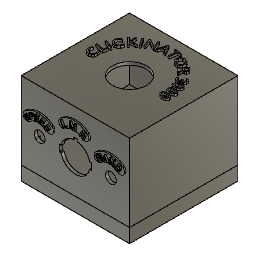
clickinator3000 v6 (Autodesk Fusion 360 design; units mm, degrees)
Autodesk Fusion 360 part; units mm, degrees
box "BoxPrimitive1" add length 70 width 70 height 50 placed x (0, 1, 0) y (-1, 0, 0) z (0, 0, 1) at (0, 0, 0) makes body 1
shell "Shell1" thickness 2 removed faces 0 bodies 1
move_body "Move1" bodies 1 to x (1, 0, 0) y (0, 1, 0) z (0, 0, 1) at (35, -35, 0)
sketch "Sketch3" plane through (0, 0, 50) normal (0, 0, 1) x (-1, 0, 0)
  line L0 (-35, -35) -> (35, -35)
  line L1 (35, -35) -> (35, 35)
  line L2 (35, 35) -> (-35, 35)
  line L3 (-35, 35) -> (-35, -35)
  circle A0 centre (0, 0) radius 11
  dimension "d7" = 22
  constraint coincident A0.centre origin
  measures "d7" diameter of A0
extrude "Extrude1" cut sketch "Sketch3" against normal up to surface (2 mm away) contours A0 bodies 1
sketch "Sketch4" plane through (0, -35, 0) normal (0, -1, 0) x (1, 0, 0)
  line L0 (-35, 50) -> (-35, 0)
  line L1 (-35, 0) -> (35, 0)
  line L2 (35, 0) -> (35, 50)
  line L3 (35, 50) -> (-35, 50)
  line L4 (0, 50) -> (0, 0) construction
  line L5 (-35, 21.8016) -> (35, 21.8016) construction
  circle A0 centre (0, 21.8016) radius 9.5
  circle A1 centre (23, 21.8016) radius 3.5
  line L6 (0, 21.8016) -> (0, 3.076) construction
  line L7 (1.1, 32.6016) -> (-1.1, 32.6016)
  line L8 (-1.1, 32.6016) -> (-1.1, 21.593)
  line L9 (-1.1, 21.593) -> (1.1, 21.593)
  line L10 (1.1, 21.593) -> (1.1, 32.6016)
  line L11 (1.1, 32.6016) -> (-1.1, 21.593) construction
  line L12 (-1.1, 32.6016) -> (1.1, 21.593) construction
  line L13 (10.4, 23.8016) -> (2.7448, 23.8016)
  line L14 (2.7448, 23.8016) -> (2.7448, 19.8016)
  line L15 (2.7448, 19.8016) -> (10.4, 19.8016)
  line L16 (10.4, 19.8016) -> (10.4, 23.8016)
  line L17 (10.4, 23.8016) -> (2.7448, 19.8016) construction
  line L18 (2.7448, 23.8016) -> (10.4, 19.8016) construction
  line L19 (0, 12.3016) -> (0, 31.3016) construction
  line L20 (-10.4, 23.8016) -> (-2.7448, 23.8016)
  line L21 (-2.7448, 19.8016) -> (-10.4, 19.8016)
  line L22 (-10.4, 19.8016) -> (-10.4, 23.8016)
  circle A2 centre (-23, 21.8016) radius 3.5
  point P0 (0, 27.0973)
  point P1 (6.5724, 21.8016)
  dimension "d10" = 19
  dimension "d12" = 7
  dimension "d14" = 2.2
  dimension "d15" = 10.8
  dimension "d16" = 4
  dimension "d17" = 10.4
  dimension "d25" = 12
  constraint midpoint L3 L4.start
  constraint coincident L4.end origin
  constraint coincident L0 L5.start
  constraint coincident L2 L5.end
  constraint perpendicular L2 L5
  constraint coincident L5 A0.centre
  constraint coincident L5 A1.centre
  constraint coincident A0.centre L6.start
  constraint perpendicular L5 L6
  constraint horizontal L7
  constraint perpendicular L7 L8
  constraint parallel L7 L9
  constraint parallel L8 L10
  constraint coincident L11 P0
  constraint coincident L12 P0
  constraint coincident L6 P0
  constraint horizontal L13
  constraint perpendicular L13 L14
  constraint parallel L13 L15
  constraint parallel L14 L16
  constraint coincident L17 P1
  constraint coincident L18 P1
  constraint coincident L5 P1
  constraint coincident L6 L19.start
  constraint coincident A0 L19.start
  constraint coincident A0 L19.end
  constraint vertical L19
  constraint symmetric L13.start L19 L20.start
  constraint symmetric L13.end L19 L20.end
  constraint symmetric L14.end L19 L21.start
  constraint symmetric L15.end L19 L21.end
  constraint coincident L4 A0.centre
  constraint symmetric L4 A1 A2
  measures "d10" diameter of A0
  measures "d12" diameter of A1
  measures "d14" distance of L8 L10
  measures "d15" distance of A0.centre L7
  measures "d16" distance of L13.end L14.end
  measures "d17" distance of A0.centre L16
  measures "d25" distance of L2 A1.centre
extrude "Extrude2" cut sketch "Sketch4" against normal up to surface (2 mm away) contours A0 L13 L14 L15 | A0 L13 L15 L16 | A0 L8 L9 L10 L13 L14 L15 | A0 L8 L9 L10 | A0 L7 L8 L10 | A0 L20 L21 L22 | A1 | A2 bodies 1
sketch "Sketch5" plane through (0, 0, 0) normal (0, 0, 1) x (1, 0, 0)
sketch "Sketch7" plane through (0, 0, 0) normal (1, 0, 0) x (0, 1, 0)
sketch "Sketch8" plane through (0, 0, 0) normal (0, 0, 1) x (1, 0, 0)
  line L0 (-22.8999, 2.8965) -> (-21.9973, 2.9285)
  spline S0 degree 2 poles (-21.9973, 2.9285) (-21.473, 2.0435) (-21.431, 0.862) knots 0 0 0 1 1 1
  spline S1 degree 2 poles (-21.431, 0.862) (-21.3969, -0.098) (-21.7588, -0.7804) knots 0 0 0 1 1 1
  spline S2 degree 2 poles (-21.7588, -0.7804) (-22.1207, -1.4628) (-22.7837, -1.8766) knots 0 0 0 1 1 1
  spline S3 degree 2 poles (-22.7837, -1.8766) (-23.4468, -2.2903) (-24.2345, -2.3183) knots 0 0 0 1 1 1
  spline S4 degree 2 poles (-24.2345, -2.3183) (-25.4857, -2.3628) (-26.3706, -1.5029) knots 0 0 0 1 1 1
  spline S5 degree 2 poles (-26.3706, -1.5029) (-27.2557, -0.6388) (-27.3022, 0.6698) knots 0 0 0 1 1 1
  spline S6 degree 2 poles (-27.3022, 0.6698) (-27.3343, 1.5724) (-26.9017, 2.6927) knots 0 0 0 1 1 1
  line L1 (-26.9017, 2.6927) -> (-26.0197, 2.724)
  spline S7 degree 2 poles (-26.0197, 2.724) (-26.5583, 1.6985) (-26.5242, 0.7386) knots 0 0 0 1 1 1
  spline S8 degree 2 poles (-26.5242, 0.7386) (-26.4892, -0.246) (-25.8425, -0.8762) knots 0 0 0 1 1 1
  spline S9 degree 2 poles (-25.8425, -0.8762) (-25.2, -1.5023) (-24.2646, -1.4691) knots 0 0 0 1 1 1
  spline S10 degree 2 poles (-24.2646, -1.4691) (-23.3211, -1.4356) (-22.7366, -0.774) knots 0 0 0 1 1 1
  spline S11 degree 2 poles (-22.7366, -0.774) (-22.1522, -0.1125) (-22.1876, 0.8844) knots 0 0 0 1 1 1
  spline S12 degree 2 poles (-22.1876, 0.8844) (-22.2246, 1.9264) (-22.8999, 2.8965) knots 0 0 0 1 1 1
  line L2 (-26.9677, 5.1045) -> (-26.8044, 5.9091)
  line L3 (-26.8044, 5.9091) -> (-21.9164, 4.9171)
  line L4 (-21.9164, 4.9171) -> (-21.4029, 7.4475)
  line L5 (-21.4029, 7.4475) -> (-20.6707, 7.2989)
  line L6 (-20.6707, 7.2989) -> (-21.3475, 3.9638)
  line L7 (-21.3475, 3.9638) -> (-26.9677, 5.1045)
  line L8 (-25.7564, 9.9218) -> (-25.4772, 10.6938)
  line L9 (-25.4772, 10.6938) -> (-20.0844, 8.7432)
  line L10 (-20.0844, 8.7432) -> (-20.3636, 7.9712)
  line L11 (-20.3636, 7.9712) -> (-25.7564, 9.9218)
  line L12 (-18.3113, 14.9034) -> (-17.536, 14.4404)
  spline S13 degree 2 poles (-17.536, 14.4404) (-17.576, 13.4124) (-18.1822, 12.3974) knots 0 0 0 1 1 1
  spline S14 degree 2 poles (-18.1822, 12.3974) (-18.6746, 11.5727) (-19.349, 11.196) knots 0 0 0 1 1 1
  spline S15 degree 2 poles (-19.349, 11.196) (-20.0233, 10.8194) (-20.8048, 10.8318) knots 0 0 0 1 1 1
  spline S16 degree 2 poles (-20.8048, 10.8318) (-21.5863, 10.8442) (-22.263, 11.2483) knots 0 0 0 1 1 1
  spline S17 degree 2 poles (-22.263, 11.2483) (-23.3379, 11.8902) (-23.6143, 13.0928) knots 0 0 0 1 1 1
  spline S18 degree 2 poles (-23.6143, 13.0928) (-23.8886, 14.2989) (-23.2173, 15.4232) knots 0 0 0 1 1 1
  spline S19 degree 2 poles (-23.2173, 15.4232) (-22.7542, 16.1986) (-21.7828, 16.9046) knots 0 0 0 1 1 1
  line L13 (-21.7828, 16.9046) -> (-21.025, 16.4521)
  spline S20 degree 2 poles (-21.025, 16.4521) (-22.0341, 15.8833) (-22.5266, 15.0586) knots 0 0 0 1 1 1
  spline S21 degree 2 poles (-22.5266, 15.0586) (-23.0317, 14.2127) (-22.8306, 13.3324) knots 0 0 0 1 1 1
  spline S22 degree 2 poles (-22.8306, 13.3324) (-22.6309, 12.4577) (-21.8273, 11.9779) knots 0 0 0 1 1 1
  spline S23 degree 2 poles (-21.8273, 11.9779) (-21.0167, 11.4938) (-20.1668, 11.7322) knots 0 0 0 1 1 1
  spline S24 degree 2 poles (-20.1668, 11.7322) (-19.3168, 11.9705) (-18.8054, 12.8269) knots 0 0 0 1 1 1
  spline S25 degree 2 poles (-18.8054, 12.8269) (-18.2708, 13.7222) (-18.3113, 14.9034) knots 0 0 0 1 1 1
  line L14 (-18.0809, 21.3843) -> (-17.3385, 22.0929)
  line L15 (-17.3385, 22.0929) -> (-17.2619, 18.4095)
  line L16 (-17.2619, 18.4095) -> (-12.9367, 18.3666)
  line L17 (-12.9367, 18.3666) -> (-13.7504, 17.59)
  line L18 (-13.7504, 17.59) -> (-17.8233, 17.6183)
  line L19 (-17.8233, 17.6183) -> (-15.8677, 15.5693)
  line L20 (-15.8677, 15.5693) -> (-16.4616, 15.0024)
  line L21 (-16.4616, 15.0024) -> (-20.421, 19.151)
  line L22 (-20.421, 19.151) -> (-19.827, 19.7178)
  line L23 (-19.827, 19.7178) -> (-18.016, 17.8202)
  line L24 (-18.016, 17.8202) -> (-18.0809, 21.3843)
  line L25 (-15.4558, 23.3953) -> (-14.7707, 23.8477)
  line L26 (-14.7707, 23.8477) -> (-11.6112, 19.0618)
  line L27 (-11.6112, 19.0618) -> (-12.2964, 18.6094)
  line L28 (-12.2964, 18.6094) -> (-15.4558, 23.3953)
  line L29 (-8.4728, 26.8725) -> (-7.7482, 27.1613)
  line L30 (-7.7482, 27.1613) -> (-5.6248, 21.8342)
  line L31 (-5.6248, 21.8342) -> (-6.2807, 21.5728)
  line L32 (-6.2807, 21.5728) -> (-11.4762, 24.2523)
  line L33 (-11.4762, 24.2523) -> (-9.8422, 20.1531)
  line L34 (-9.8422, 20.1531) -> (-10.5591, 19.8673)
  line L35 (-10.5591, 19.8673) -> (-12.6826, 25.1944)
  line L36 (-12.6826, 25.1944) -> (-12.0648, 25.4407)
  line L37 (-12.0648, 25.4407) -> (-6.8251, 22.739)
  line L38 (-6.8251, 22.739) -> (-8.4728, 26.8725)
  line L39 (-3.0804, 27.9667) -> (-2.5039, 28.0191)
  line L40 (-2.5039, 28.0191) -> (0.5733, 22.5075)
  line L41 (0.5733, 22.5075) -> (-0.2648, 22.4313)
  line L42 (-0.2648, 22.4313) -> (-1.179, 24.0547)
  line L43 (-1.179, 24.0547) -> (-3.6074, 23.8339)
  line L44 (-3.6074, 23.8339) -> (-4.1731, 22.076)
  line L45 (-4.1731, 22.076) -> (-5.0111, 21.9998)
  line L46 (-5.0111, 21.9998) -> (-3.0804, 27.9667)
  line L47 (-1.5804, 24.7519) -> (-2.6883, 26.7369)
  line L48 (-2.6883, 26.7369) -> (-3.3547, 24.5906)
  line L49 (-3.3547, 24.5906) -> (-1.5804, 24.7519)
  line L50 (1.6645, 28.1176) -> (6.394, 27.3551)
  line L51 (6.394, 27.3551) -> (6.2777, 26.6337)
  line L52 (6.2777, 26.6337) -> (4.304, 26.9519)
  line L53 (4.304, 26.9519) -> (3.5062, 22.0035)
  line L54 (3.5062, 22.0035) -> (2.6916, 22.1348)
  line L55 (2.6916, 22.1348) -> (3.4894, 27.0832)
  line L56 (3.4894, 27.0832) -> (1.5482, 27.3961)
  line L57 (1.5482, 27.3961) -> (1.6645, 28.1176)
  spline S26 degree 2 poles (11.3054, 25.5557) (12.5069, 24.9854) (12.9434, 23.8467) knots 0 0 0 1 1 1
  spline S27 degree 2 poles (12.9434, 23.8467) (13.3835, 22.7062) (12.8396, 21.5603) knots 0 0 0 1 1 1
  spline S28 degree 2 poles (12.8396, 21.5603) (12.2957, 20.4144) (11.1299, 20.0453) knots 0 0 0 1 1 1
  spline S29 degree 2 poles (11.1299, 20.0453) (9.9696, 19.6782) (8.7421, 20.2608) knots 0 0 0 1 1 1
  spline S30 degree 2 poles (8.7421, 20.2608) (7.5702, 20.8171) (7.1433, 21.9376) knots 0 0 0 1 1 1
  spline S31 degree 2 poles (7.1433, 21.9376) (6.7219, 23.0601) (7.2588, 24.1912) knots 0 0 0 1 1 1
  spline S32 degree 2 poles (7.2588, 24.1912) (7.8097, 25.3519) (8.9568, 25.739) knots 0 0 0 1 1 1
  spline S33 degree 2 poles (8.9568, 25.739) (10.1038, 26.126) (11.3054, 25.5557) knots 0 0 0 1 1 1
  spline S34 degree 2 poles (11.0006, 24.837) (10.1105, 25.2595) (9.2717, 24.9761) knots 0 0 0 1 1 1
  spline S35 degree 2 poles (9.2717, 24.9761) (8.4366, 24.6909) (8.0264, 23.8268) knots 0 0 0 1 1 1
  spline S36 degree 2 poles (8.0264, 23.8268) (7.6286, 22.9887) (7.9394, 22.1596) knots 0 0 0 1 1 1
  spline S37 degree 2 poles (7.9394, 22.1596) (8.2501, 21.3305) (9.1142, 20.9203) knots 0 0 0 1 1 1
  spline S38 degree 2 poles (9.1142, 20.9203) (9.982, 20.5084) (10.8298, 20.8012) knots 0 0 0 1 1 1
  spline S39 degree 2 poles (10.8298, 20.8012) (11.6814, 21.0923) (12.0827, 21.9378) knots 0 0 0 1 1 1
  spline S40 degree 2 poles (12.0827, 21.9378) (12.4735, 22.7611) (12.1571, 23.5974) knots 0 0 0 1 1 1
  spline S41 degree 2 poles (12.1571, 23.5974) (11.8461, 24.4357) (11.0006, 24.837) knots 0 0 0 1 1 1
  line L58 (12.4066, 18.2385) -> (16.2174, 22.5238)
  line L59 (16.2174, 22.5238) -> (17.2911, 21.5691)
  spline S42 degree 2 poles (17.2911, 21.5691) (17.9414, 20.9908) (18.0353, 20.3304) knots 0 0 0 1 1 1
  spline S43 degree 2 poles (18.0353, 20.3304) (18.1324, 19.6673) (17.6441, 19.1182) knots 0 0 0 1 1 1
  spline S44 degree 2 poles (17.6441, 19.1182) (17.3113, 18.744) (16.8814, 18.6374) knots 0 0 0 1 1 1
  spline S45 degree 2 poles (16.8814, 18.6374) (16.4515, 18.5308) (15.9817, 18.7067) knots 0 0 0 1 1 1
  spline S46 degree 2 poles (15.9817, 18.7067) (16.0672, 18.389) (16.0562, 17.9813) knots 0 0 0 1 1 1
  spline S47 degree 2 poles (16.0562, 17.9813) (16.0452, 17.5735) (15.8855, 16.6773) knots 0 0 0 1 1 1
  spline S48 degree 2 poles (15.8855, 16.6773) (15.7848, 16.1132) (15.7561, 15.8091) knots 0 0 0 1 1 1
  line L60 (15.7561, 15.8091) -> (15.7103, 15.3005)
  line L61 (15.7103, 15.3005) -> (14.9802, 15.9497)
  line L62 (14.9802, 15.9497) -> (15.0441, 16.3983)
  spline S49 degree 2 poles (15.0441, 16.3983) (15.0485, 16.4218) (15.0537, 16.4832) knots 0 0 0 1 1 1
  line L63 (15.0537, 16.4832) -> (15.0841, 16.7583)
  line L64 (15.0841, 16.7583) -> (15.1721, 17.2403)
  line L65 (15.1721, 17.2403) -> (15.2639, 17.7575)
  spline S50 degree 2 poles (15.2639, 17.7575) (15.3083, 18.1904) (15.2879, 18.4887) knots 0 0 0 1 1 1
  spline S51 degree 2 poles (15.2879, 18.4887) (15.2706, 18.7843) (15.2018, 18.9663) knots 0 0 0 1 1 1
  spline S52 degree 2 poles (15.2018, 18.9663) (15.1388, 19.1487) (14.8382, 19.4161) knots 0 0 0 1 1 1
  line L66 (14.8382, 19.4161) -> (14.6786, 19.5579)
  line L67 (14.6786, 19.5579) -> (13.0201, 17.6928)
  line L68 (13.0201, 17.6928) -> (12.4066, 18.2385)
  line L69 (16.5513, 21.2931) -> (16.3672, 21.4568)
  line L70 (16.3672, 21.4568) -> (15.1642, 20.104)
  line L71 (15.1642, 20.104) -> (15.3973, 19.8967)
  spline S53 degree 2 poles (15.3973, 19.8967) (15.8636, 19.482) (16.1063, 19.409) knots 0 0 0 1 1 1
  spline S54 degree 2 poles (16.1063, 19.409) (16.3521, 19.3332) (16.589, 19.4082) knots 0 0 0 1 1 1
  spline S55 degree 2 poles (16.589, 19.4082) (16.8318, 19.4835) (17.0145, 19.689) knots 0 0 0 1 1 1
  spline S56 degree 2 poles (17.0145, 19.689) (17.1946, 19.8915) (17.2318, 20.1495) knots 0 0 0 1 1 1
  spline S57 degree 2 poles (17.2318, 20.1495) (17.2717, 20.4107) (17.1354, 20.6527) knots 0 0 0 1 1 1
  spline S58 degree 2 poles (17.1354, 20.6527) (17.0022, 20.8921) (16.5513, 21.2931) knots 0 0 0 1 1 1
  line L72 (20.7885, 13.7546) -> (20.8128, 13.7118)
  spline S59 degree 2 poles (20.8128, 13.7118) (21.0786, 13.2443) (21.4092, 13.1112) knots 0 0 0 1 1 1
  spline S60 degree 2 poles (21.4092, 13.1112) (21.7419, 12.9745) (22.1095, 13.1835) knots 0 0 0 1 1 1
  spline S61 degree 2 poles (22.1095, 13.1835) (22.4414, 13.3721) (22.5124, 13.7289) knots 0 0 0 1 1 1
  spline S62 degree 2 poles (22.5124, 13.7289) (22.5855, 14.0821) (22.3664, 14.4675) knots 0 0 0 1 1 1
  spline S63 degree 2 poles (22.3664, 14.4675) (22.1453, 14.8565) (21.6328, 15.1932) knots 0 0 0 1 1 1
  line L73 (21.6328, 15.1932) -> (22.3144, 15.5807)
  spline S64 degree 2 poles (22.3144, 15.5807) (22.7796, 15.269) (23.0718, 14.7552) knots 0 0 0 1 1 1
  spline S65 degree 2 poles (23.0718, 14.7552) (23.4633, 14.0664) (23.3281, 13.4654) knots 0 0 0 1 1 1
  spline S66 degree 2 poles (23.3281, 13.4654) (23.1948, 12.8608) (22.5703, 12.5058) knots 0 0 0 1 1 1
  spline S67 degree 2 poles (22.5703, 12.5058) (22.192, 12.2907) (21.8443, 12.2961) knots 0 0 0 1 1 1
  spline S68 degree 2 poles (21.8443, 12.2961) (21.5001, 12.3035) (21.1238, 12.5334) knots 0 0 0 1 1 1
  spline S69 degree 2 poles (21.1238, 12.5334) (21.176, 12.1759) (21.0853, 11.9449) knots 0 0 0 1 1 1
  spline S70 degree 2 poles (21.0853, 11.9449) (20.9983, 11.716) (20.8053, 11.5071) knots 0 0 0 1 1 1
  spline S71 degree 2 poles (20.8053, 11.5071) (20.6124, 11.2983) (20.3483, 11.1482) knots 0 0 0 1 1 1
  spline S72 degree 2 poles (20.3483, 11.1482) (19.6953, 10.7769) (19.0195, 10.9688) knots 0 0 0 1 1 1
  spline S73 degree 2 poles (19.0195, 10.9688) (18.3473, 11.1628) (17.97, 11.8266) knots 0 0 0 1 1 1
  spline S74 degree 2 poles (17.97, 11.8266) (17.6474, 12.394) (17.622, 13.0784) knots 0 0 0 1 1 1
  line L74 (17.622, 13.0784) -> (18.3999, 13.5206)
  spline S75 degree 2 poles (18.3999, 13.5206) (18.3672, 12.7559) (18.6695, 12.2242) knots 0 0 0 1 1 1
  spline S76 degree 2 poles (18.6695, 12.2242) (18.8744, 11.8638) (19.2122, 11.7678) knots 0 0 0 1 1 1
  spline S77 degree 2 poles (19.2122, 11.7678) (19.5521, 11.6682) (19.9054, 11.8691) knots 0 0 0 1 1 1
  spline S78 degree 2 poles (19.9054, 11.8691) (20.2016, 12.0375) (20.3194, 12.3453) knots 0 0 0 1 1 1
  spline S79 degree 2 poles (20.3194, 12.3453) (20.3835, 12.5233) (20.3655, 12.6878) knots 0 0 0 1 1 1
  spline S80 degree 2 poles (20.3655, 12.6878) (20.3531, 12.8508) (20.1611, 13.313) knots 0 0 0 1 1 1
  line L75 (20.1611, 13.313) -> (20.1318, 13.3813)
  line L76 (20.1318, 13.3813) -> (20.7885, 13.7546)
  spline S81 degree 2 poles (25.4073, 9.5475) (25.6541, 8.799) (25.0274, 8.052) knots 0 0 0 1 1 1
  spline S82 degree 2 poles (25.0274, 8.052) (24.4058, 7.3023) (23.1972, 6.9038) knots 0 0 0 1 1 1
  spline S83 degree 2 poles (23.1972, 6.9038) (21.9575, 6.4949) (21.0197, 6.7303) knots 0 0 0 1 1 1
  spline S84 degree 2 poles (21.0197, 6.7303) (20.0832, 6.9617) (19.8261, 7.7414) knots 0 0 0 1 1 1
  spline S85 degree 2 poles (19.8261, 7.7414) (19.5651, 8.5328) (20.1671, 9.263) knots 0 0 0 1 1 1
  spline S86 degree 2 poles (20.1671, 9.263) (20.7692, 9.9933) (22.0245, 10.4073) knots 0 0 0 1 1 1
  spline S87 degree 2 poles (22.0245, 10.4073) (23.2642, 10.8161) (24.2033, 10.5769) knots 0 0 0 1 1 1
  spline S88 degree 2 poles (24.2033, 10.5769) (25.1463, 10.3389) (25.4073, 9.5475) knots 0 0 0 1 1 1
  line L77 (24.6691, 9.2954) -> (24.6563, 9.3344)
  spline S89 degree 2 poles (24.6563, 9.3344) (24.5084, 9.7828) (23.8674, 9.8653) knots 0 0 0 1 1 1
  spline S90 degree 2 poles (23.8674, 9.8653) (23.2316, 9.9452) (22.2881, 9.6341) knots 0 0 0 1 1 1
  spline S91 degree 2 poles (22.2881, 9.6341) (21.3213, 9.3152) (20.8565, 8.8766) knots 0 0 0 1 1 1
  spline S92 degree 2 poles (20.8565, 8.8766) (20.3917, 8.438) (20.5408, 7.9858) knots 0 0 0 1 1 1
  spline S93 degree 2 poles (20.5408, 7.9858) (20.69, 7.5336) (21.3258, 7.4537) knots 0 0 0 1 1 1
  spline S94 degree 2 poles (21.3258, 7.4537) (21.9616, 7.3738) (22.905, 7.6849) knots 0 0 0 1 1 1
  spline S95 degree 2 poles (22.905, 7.6849) (23.8524, 7.9973) (24.3302, 8.4359) knots 0 0 0 1 1 1
  spline S96 degree 2 poles (24.3302, 8.4359) (24.8093, 8.8705) (24.6691, 9.2954) knots 0 0 0 1 1 1
  spline S97 degree 2 poles (26.5632, 4.3205) (26.6568, 3.5379) (25.8945, 2.9298) knots 0 0 0 1 1 1
  spline S98 degree 2 poles (25.8945, 2.9298) (25.1367, 2.3182) (23.8731, 2.167) knots 0 0 0 1 1 1
  spline S99 degree 2 poles (23.8731, 2.167) (22.577, 2.0119) (21.7044, 2.4284) knots 0 0 0 1 1 1
  spline S100 degree 2 poles (21.7044, 2.4284) (20.8323, 2.8408) (20.7348, 3.656) knots 0 0 0 1 1 1
  spline S101 degree 2 poles (20.7348, 3.656) (20.6357, 4.4834) (21.3706, 5.0799) knots 0 0 0 1 1 1
  spline S102 degree 2 poles (21.3706, 5.0799) (22.1054, 5.6764) (23.4178, 5.8334) knots 0 0 0 1 1 1
  spline S103 degree 2 poles (23.4178, 5.8334) (24.714, 5.9886) (25.587, 5.568) knots 0 0 0 1 1 1
  spline S104 degree 2 poles (25.587, 5.568) (26.4642, 5.1479) (26.5632, 4.3205) knots 0 0 0 1 1 1
  line L78 (25.7897, 4.2196) -> (25.7848, 4.2604)
  spline S105 degree 2 poles (25.7848, 4.2604) (25.7287, 4.7291) (25.1168, 4.9371) knots 0 0 0 1 1 1
  spline S106 degree 2 poles (25.1168, 4.9371) (24.5094, 5.1414) (23.523, 5.0234) knots 0 0 0 1 1 1
  spline S107 degree 2 poles (23.523, 5.0234) (22.5122, 4.9024) (21.9697, 4.5646) knots 0 0 0 1 1 1
  spline S108 degree 2 poles (21.9697, 4.5646) (21.4272, 4.2268) (21.4837, 3.754) knots 0 0 0 1 1 1
  spline S109 degree 2 poles (21.4837, 3.754) (21.5403, 3.2812) (22.1477, 3.0769) knots 0 0 0 1 1 1
  spline S110 degree 2 poles (22.1477, 3.0769) (22.7551, 2.8726) (23.7415, 2.9906) knots 0 0 0 1 1 1
  spline S111 degree 2 poles (23.7415, 2.9906) (24.7319, 3.1091) (25.2872, 3.4443) knots 0 0 0 1 1 1
  spline S112 degree 2 poles (25.2872, 3.4443) (25.8429, 3.7754) (25.7897, 4.2196) knots 0 0 0 1 1 1
  spline S113 degree 2 poles (26.663, -1.0225) (26.601, -1.8083) (25.734, -2.2546) knots 0 0 0 1 1 1
  spline S114 degree 2 poles (25.734, -2.2546) (24.8707, -2.7053) (23.6021, -2.6052) knots 0 0 0 1 1 1
  spline S115 degree 2 poles (23.6021, -2.6052) (22.3008, -2.5026) (21.5271, -1.9227) knots 0 0 0 1 1 1
  spline S116 degree 2 poles (21.5271, -1.9227) (20.7531, -1.3469) (20.8176, -0.5285) knots 0 0 0 1 1 1
  spline S117 degree 2 poles (20.8176, -0.5285) (20.8832, 0.3023) (21.7209, 0.7427) knots 0 0 0 1 1 1
  spline S118 degree 2 poles (21.7209, 0.7427) (22.5586, 1.1831) (23.8763, 1.0791) knots 0 0 0 1 1 1
  spline S119 degree 2 poles (23.8763, 1.0791) (25.1777, 0.9765) (25.951, 0.3925) knots 0 0 0 1 1 1
  spline S120 degree 2 poles (25.951, 0.3925) (26.7285, -0.1918) (26.663, -1.0225) knots 0 0 0 1 1 1
  line L79 (25.8848, -0.9694) -> (25.888, -0.9284)
  spline S121 degree 2 poles (25.888, -0.9284) (25.9252, -0.4578) (25.366, -0.1337) knots 0 0 0 1 1 1
  spline S122 degree 2 poles (25.366, -0.1337) (24.8106, 0.186) (23.8203, 0.2642) knots 0 0 0 1 1 1
  spline S123 degree 2 poles (23.8203, 0.2642) (22.8054, 0.3443) (22.2071, 0.1197) knots 0 0 0 1 1 1
  spline S124 degree 2 poles (22.2071, 0.1197) (21.6087, -0.1049) (21.5713, -0.5796) knots 0 0 0 1 1 1
  spline S125 degree 2 poles (21.5713, -0.5796) (21.5338, -1.0543) (22.0892, -1.374) knots 0 0 0 1 1 1
  spline S126 degree 2 poles (22.0892, -1.374) (22.6446, -1.6937) (23.635, -1.7718) knots 0 0 0 1 1 1
  spline S127 degree 2 poles (23.635, -1.7718) (24.6294, -1.8503) (25.2397, -1.6308) knots 0 0 0 1 1 1
  spline S128 degree 2 poles (25.2397, -1.6308) (25.8496, -1.4153) (25.8848, -0.9694) knots 0 0 0 1 1 1
sketch "Sketch9" plane through (0, 0, 50) normal (0, 0, 1) x (-1, 0, 0)
  circle A0 centre (0, 0) radius 11
  line L0 (-35, -35) -> (35, -35)
  line L1 (35, -35) -> (35, 35)
  line L2 (35, 35) -> (-35, 35)
  line L3 (-35, 35) -> (-35, -35)
emboss "Emboss1" depth 1.4 profiles "Sketch8" section 1 onto face at (0.274, -26.9897, 50) on bodies 1 bodies 1
sketch "Sketch11" plane through (0, 0, 0) normal (0, 0, -1) x (1, 0, 0)
  line L0 (-35, -35) -> (35, -35)
  line L1 (35, -35) -> (35, 35)
  line L2 (35, 35) -> (-35, 35)
  line L3 (-35, 35) -> (-35, -35)
  line L4 (35, 35) -> (-35, 35)
  line L5 (-35, 35) -> (-35, -35)
  line L6 (35, -35) -> (35, 35)
  line L7 (-35, -35) -> (35, -35)
  line L8 (-35, 35) -> (35, 35)
  line L9 (35, 35) -> (35, -35)
  line L10 (35, -35) -> (-35, -35)
  line L11 (-35, -35) -> (-35, 35)
  line L12 (-33, -33) -> (-33, 33)
  line L13 (-33, 33) -> (33, 33)
  line L14 (33, 33) -> (33, -33)
  line L15 (33, -33) -> (-33, -33)
  line L16 (-33, 24.2087) -> (-24.2087, 33)
  line L17 (-33, 24.2087) -> (-20.5081, 24.2087) construction
  line L18 (0, -1.75) -> (0, -22.5)
  line L19 (33, 24.2087) -> (24.2087, 33)
  line L20 (1.75, 0) -> (22.5, 0)
  line L21 (-33, -24.2087) -> (-24.2087, -33)
  line L22 (33, -24.2087) -> (24.2087, -33)
  dimension "d26" = 2
  dimension "d29" = 45
  constraint horizontal L8
  constraint vertical L9
  constraint horizontal L10
  constraint vertical L11
  constraint coincident L0.end L1.start
  constraint coincident L2.end L3.start
  constraint horizontal L17
  constraint coincident L12 L16.start
  constraint coincident L13 L16.end
  constraint symmetric L16.start L18 L19.start
  constraint symmetric L16.end L18 L19.end
  constraint symmetric L16.start L20 L21.start
  constraint symmetric L16.end L20 L21.end
  constraint symmetric L19.start L20 L22.start
  constraint symmetric L19.end L20 L22.end
  measures "d29" angle of L16 L17
extrude "Extrude3" cut sketch "Sketch11" against normal blind 2 contours L12 L15 L21 | L12 L13 L14 L15 L16 L19 L21 L22 | L12 L13 L16 | L14 L15 L22 | L13 L14 L19 bodies 1
ref_plane "WorkPlane1" through (0, 0, 2) normal (0, 0, 1) x (1, 0, 0)
sketch "Sketch14" plane through (0, 0, 2) normal (0, 0, 1) x (1, 0, 0)
  line L0 (33, 33) -> (-33, 33)
  line L1 (33, 24.2087) -> (24.2087, 33)
  line L2 (33, -33) -> (33, 33)
  line L3 (-33, 24.2087) -> (-24.2087, 33)
  line L4 (-33, 33) -> (-33, -33)
  line L5 (-33, -33) -> (33, -33)
  line L6 (-33, -24.2087) -> (-24.2087, -33)
  line L7 (33, -24.2087) -> (24.2087, -33)
  circle A0 centre (-30.5589, -30.5589) radius 1.9
  line L8 (0, 1.75) -> (0, 22.5)
  circle A1 centre (30.5589, -30.5589) radius 1.9
  line L9 (1.75, 0) -> (22.5, 0)
  circle A2 centre (-30.5589, 30.5589) radius 1.9
  circle A3 centre (30.5589, 30.5589) radius 1.9
  dimension "d35" = 3.8
  constraint symmetric A0 L8 A1
  constraint symmetric A0 L9 A2
  constraint symmetric A1 L9 A3
  measures "d35" diameter of A0
extrude "Extrude5" add sketch "Sketch14" along normal blind 10 contours L0 L1 L2 | L0 L3 L4 | L2 L5 L7 | L4 L5 L6 | A0 | A1 | A2 | A3 bodies 1
extrude "Extrude6" cut sketch "Sketch14" along normal blind 7 contours A0 | A1 | A2 | A3 bodies 1
sketch "Sketch1" plane through (0, 0, 0) normal (0, 0, 1) x (1, 0, 0) in component "base"
  circle A0 centre (-30.5589, -30.5589) radius 1.9
  circle A1 centre (30.5589, -30.5589) radius 1.9
  circle A2 centre (-30.5589, 30.5589) radius 1.9
  circle A3 centre (30.5589, 30.5589) radius 1.9
  line L0 (-35, -35) -> (35, -35)
  line L1 (35, -35) -> (35, 35)
  line L2 (35, 35) -> (-35, 35)
  line L3 (-35, 35) -> (-35, -35)
  line L4 (-32.7, -32.7) -> (32.7, -32.7)
  line L5 (32.7, -32.7) -> (32.7, 32.7)
  line L6 (32.7, 32.7) -> (-32.7, 32.7)
  line L7 (-32.7, 32.7) -> (-32.7, -32.7)
  line L8 (0, 35) -> (0, -35) construction
  line L9 (-10, 35) -> (10, 35) construction
  line L10 (10, 35) -> (10, -5)
  line L11 (10, -5) -> (-10, -5)
  line L12 (-10, -5) -> (-10, 35)
  circle A4 centre (-30.5589, -30.5589) radius 1.55
  circle A5 centre (30.5589, -30.5589) radius 1.9
  circle A6 centre (-30.5589, 30.5589) radius 1.55
  circle A7 centre (30.5589, 30.5589) radius 1.55
  circle A8 centre (30.5589, -30.5589) radius 1.55
  point P0 (-35, -35)
  point P1 (35, -35)
  point P2 (35, 35)
  point P3 (-35, 35)
  point P4 (-33, 33)
  point P5 (-33, -33)
  point P6 (33, -33)
  point P7 (33, 33)
  dimension "d38" = -2.3
  dimension "d41" = 20
  dimension "d42" = 40
  dimension "d43" = 10
  dimension "d53" = 3.1
  dimension "d54" = 3.1
  dimension "d55" = 3.1
  dimension "d56" = 3.1
  constraint horizontal L0
  constraint vertical L1
  constraint horizontal L2
  constraint vertical L3
  constraint coincident P2 L1.end
  constraint coincident P0 L0.start
  constraint midpoint L2 L8.start
  constraint midpoint L0 L8.end
  constraint horizontal L9
  constraint vertical L10
  constraint horizontal L11
  constraint vertical L12
  constraint coincident L2 L9.start
  constraint concentric A0 A4
  constraint concentric A2 A6
  constraint concentric A3 A7
  constraint concentric A1 A8
  measures "d41" distance of L9.start L9.end
  measures "d42" distance of L9.start L11.end
  measures "d43" distance of L8 L10
  measures "d53" diameter of A4
  measures "d54" diameter of A6
  measures "d55" diameter of A7
  measures "d56" diameter of A8
extrude "Extrude1'" add sketch "Sketch1" along normal blind 1.6 separate body contours A0 | A1 A5 | A2 | A3 | L4 L5 L6 L7 L10 L11 L12 makes body 2 in component "base"
extrude "Extrude2'" add sketch "Sketch1" against normal blind 7 contours A0 | A1 A5 | A2 | A3 | L0 L1 L2 L3 L4 L5 L6 L7 L10 L12 | L2 L6 L10 L12 | L4 L5 L6 L7 L10 L11 L12 bodies 2 in component "base"
sketch "Sketch2" plane through (0, 35, 0) normal (0, 1, 0) x (-1, 0, 0) in component "base"
  line L0 (35, 0) -> (-35, 0)
  line L1 (-35, 0) -> (-35, -7)
  line L2 (-35, -7) -> (35, -7)
  line L3 (35, -7) -> (35, 0)
  line L4 (-2.85, -3.5) -> (2.85, -3.5)
  arc A0 (2.85, -3.5) -> (2.85, 0) centre (2.85, -1.75) ccw
  line L5 (2.85, 0) -> (-2.85, 0)
  arc A1 (-2.85, 0) -> (-2.85, -3.5) centre (-2.85, -1.75) ccw
  line L6 (16.6901, 0) -> (25.8901, 0) construction
  line L7 (-35, 0) -> (35, 0)
  dimension "d46" = 9.2
  dimension "d47" = 3.5
  constraint tangent L4 A0
  constraint tangent A0 L5
  constraint parallel L4 L5
  constraint tangent L5 A1
  constraint tangent L4 A1
  constraint parallel L0 L6
  constraint coincident L0 L6.start
  constraint horizontal L5
  constraint coincident L5.end L7
  constraint midpoint L5 L7
  measures "d46" distance of L6.start L6.end
  measures "d47" distance of L4 L5
extrude "Extrude3'" cut sketch "Sketch2" against normal up to surface (2.3 mm away) contours L0 L4 A0 L5 A1 L7 bodies 2 in component "base"
extrude "Extrude4" add sketch "Sketch1" against normal blind 2 from surface at -7 contours A0 | A1 A5 | A2 | A3 | L0 L1 L2 L3 L4 L5 L6 L7 L10 L12 | L2 L6 L10 L12 | L4 L5 L6 L7 L10 L11 L12 | L6 L10 L11 L12 bodies 2 in component "base"
fillet "Fillet1" radius 0.8 4 edges at (-32.004, -31.1194, -9) (29.1138, -31.1194, -9) (-32.004, 29.9984, -9) (29.1138, 29.9984, -9) on bodies 2 in component "base"
sketch "Sketch1 (2)" plane through (0, -35, 0) normal (0, -1, 0) x (1, 0, 0) in component "dials"
  line L0 (-1.1, 31.2377) -> (-1.1, 32.6016)
  line L1 (-1.1, 32.6016) -> (1.1, 32.6016)
  line L2 (1.1, 32.6016) -> (1.1, 31.2377)
  arc A0 (9.2871, 23.8016) -> (1.1, 31.2377) centre (0, 21.8016) ccw
  line L3 (9.2871, 23.8016) -> (10.4, 23.8016)
  line L4 (10.4, 23.8016) -> (10.4, 19.8016)
  line L5 (10.4, 19.8016) -> (9.2871, 19.8016)
  arc A1 (-9.2871, 19.8016) -> (9.2871, 19.8016) centre (0, 21.8016) ccw
  line L6 (-9.2871, 19.8016) -> (-10.4, 19.8016)
  line L7 (-10.4, 19.8016) -> (-10.4, 23.8016)
  line L8 (-10.4, 23.8016) -> (-9.2871, 23.8016)
  arc A2 (-1.1, 31.2377) -> (-9.2871, 23.8016) centre (0, 21.8016) ccw
  circle A3 centre (23, 21.8016) radius 3.5
  line L9 (-35, 50) -> (-35, 0)
  line L10 (-35, 0) -> (35, 0)
  line L11 (35, 0) -> (35, 50)
  line L12 (35, 50) -> (-35, 50)
  circle A4 centre (-23, 21.8016) radius 7.5 construction
  circle A5 centre (-22.9916, 21.8016) radius 7.5 construction
  arc A6 (-14.1652, 32.3404) -> (-31.818, 32.3404) centre (-22.9916, 21.8016) ccw
  arc A7 (-17.6176, 28.2182) -> (-14.1652, 32.3404) centre (-15.8914, 30.2793) ccw
  arc A8 (-17.6176, 28.2182) -> (-28.3656, 28.2182) centre (-22.9916, 21.8016) ccw
  arc A9 (-31.818, 32.3404) -> (-28.3656, 28.2182) centre (-30.0918, 30.2793) ccw
  arc A10 (-15.8914, 30.2793) -> (-30.0918, 30.2793) centre (-22.9916, 21.8016) ccw construction
  spline S0 degree 2 poles (-29.9147, 29.488) (-29.7283, 29.2947) (-29.5346, 29.2409) knots 0 0 0 1 1 1
  spline S1 degree 2 poles (-29.5346, 29.2409) (-29.1693, 29.1424) (-28.7633, 29.4925) knots 0 0 0 1 1 1
  spline S2 degree 2 poles (-28.7633, 29.4925) (-28.5813, 29.6493) (-28.4767, 29.8301) knots 0 0 0 1 1 1
  spline S3 degree 2 poles (-28.4767, 29.8301) (-28.2744, 30.1801) (-28.4985, 30.44) knots 0 0 0 1 1 1
  spline S4 degree 2 poles (-28.4985, 30.44) (-28.6665, 30.6349) (-28.8598, 30.6127) knots 0 0 0 1 1 1
  spline S5 degree 2 poles (-28.8598, 30.6127) (-29.0532, 30.5875) (-29.3682, 30.4207) knots 0 0 0 1 1 1
  line L13 (-29.3682, 30.4207) -> (-29.7544, 30.2151)
  spline S6 degree 2 poles (-29.7544, 30.2151) (-30.1328, 30.0135) (-30.3385, 29.9862) knots 0 0 0 1 1 1
  spline S7 degree 2 poles (-30.3385, 29.9862) (-30.6948, 29.9395) (-30.951, 30.2368) knots 0 0 0 1 1 1
  spline S8 degree 2 poles (-30.951, 30.2368) (-31.2283, 30.5584) (-31.1836, 30.9565) knots 0 0 0 1 1 1
  spline S9 degree 2 poles (-31.1836, 30.9565) (-31.139, 31.3547) (-30.7313, 31.7061) knots 0 0 0 1 1 1
  spline S10 degree 2 poles (-30.7313, 31.7061) (-30.3561, 32.0296) (-29.9377, 32.0732) knots 0 0 0 1 1 1
  spline S11 degree 2 poles (-29.9377, 32.0732) (-29.5192, 32.1197) (-29.1761, 31.7218) knots 0 0 0 1 1 1
  line L14 (-29.1761, 31.7218) -> (-29.4798, 31.4599)
  spline S12 degree 2 poles (-29.4798, 31.4599) (-29.6694, 31.6306) (-29.8372, 31.6643) knots 0 0 0 1 1 1
  spline S13 degree 2 poles (-29.8372, 31.6643) (-30.1461, 31.7237) (-30.5002, 31.4184) knots 0 0 0 1 1 1
  spline S14 degree 2 poles (-30.5002, 31.4184) (-30.786, 31.1719) (-30.8075, 30.9439) knots 0 0 0 1 1 1
  spline S15 degree 2 poles (-30.8075, 30.9439) (-30.8289, 30.7159) (-30.6917, 30.5567) knots 0 0 0 1 1 1
  spline S16 degree 2 poles (-30.6917, 30.5567) (-30.5404, 30.3813) (-30.3242, 30.4261) knots 0 0 0 1 1 1
  spline S17 degree 2 poles (-30.3242, 30.4261) (-30.1836, 30.4567) (-29.7785, 30.67) knots 0 0 0 1 1 1
  line L15 (-29.7785, 30.67) -> (-29.3781, 30.8822)
  spline S18 degree 2 poles (-29.3781, 30.8822) (-29.0885, 31.0356) (-28.8743, 31.0532) knots 0 0 0 1 1 1
  spline S19 degree 2 poles (-28.8743, 31.0532) (-28.5027, 31.082) (-28.2282, 30.7636) knots 0 0 0 1 1 1
  spline S20 degree 2 poles (-28.2282, 30.7636) (-27.8865, 30.3673) (-28.0286, 29.9475) knots 0 0 0 1 1 1
  spline S21 degree 2 poles (-28.0286, 29.9475) (-28.169, 29.5291) (-28.5507, 29.2) knots 0 0 0 1 1 1
  spline S22 degree 2 poles (-28.5507, 29.2) (-28.9958, 28.8163) (-29.4436, 28.8266) knots 0 0 0 1 1 1
  spline S23 degree 2 poles (-29.4436, 28.8266) (-29.89, 28.8353) (-30.2184, 29.2261) knots 0 0 0 1 1 1
  line L16 (-30.2184, 29.2261) -> (-29.9147, 29.488)
  line L17 (-28.2359, 33.3282) -> (-26.9106, 33.8313)
  spline S24 degree 2 poles (-26.9106, 33.8313) (-26.5176, 33.9805) (-26.1925, 33.8493) knots 0 0 0 1 1 1
  spline S25 degree 2 poles (-26.1925, 33.8493) (-25.8682, 33.72) (-25.716, 33.319) knots 0 0 0 1 1 1
  spline S26 degree 2 poles (-25.716, 33.319) (-25.5851, 32.9742) (-25.7022, 32.6361) knots 0 0 0 1 1 1
  spline S27 degree 2 poles (-25.7022, 32.6361) (-25.8201, 32.3) (-26.2652, 32.1311) knots 0 0 0 1 1 1
  line L18 (-26.2652, 32.1311) -> (-27.1915, 31.7794)
  line L19 (-27.1915, 31.7794) -> (-26.7189, 30.5343)
  line L20 (-26.7189, 30.5343) -> (-27.1179, 30.3829)
  line L21 (-27.1179, 30.3829) -> (-28.2359, 33.3282)
  spline S28 degree 2 poles (-26.1182, 33.1641) (-26.2415, 33.4889) (-26.5263, 33.5138) knots 0 0 0 1 1 1
  spline S29 degree 2 poles (-26.5263, 33.5138) (-26.6822, 33.5257) (-26.9128, 33.4382) knots 0 0 0 1 1 1
  line L22 (-26.9128, 33.4382) -> (-27.7067, 33.1368)
  line L23 (-27.7067, 33.1368) -> (-27.3194, 32.1163)
  line L24 (-27.3194, 32.1163) -> (-26.5254, 32.4177)
  spline S30 degree 2 poles (-26.5254, 32.4177) (-26.2567, 32.5197) (-26.1337, 32.6971) knots 0 0 0 1 1 1
  spline S31 degree 2 poles (-26.1337, 32.6971) (-26.0086, 32.8753) (-26.1182, 33.1641) knots 0 0 0 1 1 1
  line L25 (-24.3658, 34.4496) -> (-22.0692, 34.4822)
  line L26 (-22.0692, 34.4822) -> (-22.0637, 34.0962)
  line L27 (-22.0637, 34.0962) -> (-23.9443, 34.0696)
  line L28 (-23.9443, 34.0696) -> (-23.9308, 33.1132)
  line L29 (-23.9308, 33.1132) -> (-22.1917, 33.1378)
  line L30 (-22.1917, 33.1378) -> (-22.1865, 32.7733)
  line L31 (-22.1865, 32.7733) -> (-23.9256, 32.7486)
  line L32 (-23.9256, 32.7486) -> (-23.9105, 31.6807)
  line L33 (-23.9105, 31.6807) -> (-21.9977, 31.7078)
  line L34 (-21.9977, 31.7078) -> (-21.9924, 31.3326)
  line L35 (-21.9924, 31.3326) -> (-24.3212, 31.2996)
  line L36 (-24.3212, 31.2996) -> (-24.3658, 34.4496)
  line L37 (-20.3458, 34.1865) -> (-18.1759, 33.4333)
  line L38 (-18.1759, 33.4333) -> (-18.3025, 33.0686)
  line L39 (-18.3025, 33.0686) -> (-20.0793, 33.6853)
  line L40 (-20.0793, 33.6853) -> (-20.3929, 32.7817)
  line L41 (-20.3929, 32.7817) -> (-18.7499, 32.2114)
  line L42 (-18.7499, 32.2114) -> (-18.8694, 31.867)
  line L43 (-18.8694, 31.867) -> (-20.5125, 32.4373)
  line L44 (-20.5125, 32.4373) -> (-20.8627, 31.4284)
  line L45 (-20.8627, 31.4284) -> (-19.0555, 30.8011)
  line L46 (-19.0555, 30.8011) -> (-19.1786, 30.4465)
  line L47 (-19.1786, 30.4465) -> (-21.3788, 31.2103)
  line L48 (-21.3788, 31.2103) -> (-20.3458, 34.1865)
  spline S32 degree 2 poles (-17.505, 29.6602) (-17.3389, 29.5211) (-17.2032, 29.4661) knots 0 0 0 1 1 1
  spline S33 degree 2 poles (-17.2032, 29.4661) (-16.9587, 29.3705) (-16.6842, 29.4511) knots 0 0 0 1 1 1
  spline S34 degree 2 poles (-16.6842, 29.4511) (-16.4647, 29.5162) (-16.2305, 29.7089) knots 0 0 0 1 1 1
  spline S35 degree 2 poles (-16.2305, 29.7089) (-16.0915, 29.8247) (-15.9938, 29.9414) knots 0 0 0 1 1 1
  spline S36 degree 2 poles (-15.9938, 29.9414) (-15.6178, 30.3902) (-15.589, 30.7886) knots 0 0 0 1 1 1
  spline S37 degree 2 poles (-15.589, 30.7886) (-15.5587, 31.1855) (-15.9549, 31.5174) knots 0 0 0 1 1 1
  line L49 (-15.9549, 31.5174) -> (-16.5352, 32.0035)
  line L50 (-16.5352, 32.0035) -> (-18.0886, 30.1491)
  line L51 (-18.0886, 30.1491) -> (-17.505, 29.6602)
  line L52 (-16.6285, 32.5601) -> (-15.6503, 31.7407)
  spline S38 degree 2 poles (-15.6503, 31.7407) (-15.1522, 31.3234) (-15.1737, 30.74) knots 0 0 0 1 1 1
  spline S39 degree 2 poles (-15.1737, 30.74) (-15.1959, 30.2159) (-15.6132, 29.7177) knots 0 0 0 1 1 1
  spline S40 degree 2 poles (-15.6132, 29.7177) (-15.9354, 29.333) (-16.3404, 29.1435) knots 0 0 0 1 1 1
  spline S41 degree 2 poles (-16.3404, 29.1435) (-17.0552, 28.8079) (-17.6766, 29.3284) knots 0 0 0 1 1 1
  line L53 (-17.6766, 29.3284) -> (-18.6515, 30.145)
  line L54 (-18.6515, 30.145) -> (-16.6285, 32.5601)
  arc A11 (28.2966, 28.2182) -> (31.749, 32.3404) centre (30.0228, 30.2793) ccw
  arc A12 (31.749, 32.3404) -> (14.0962, 32.3404) centre (22.9226, 21.8016) ccw
  arc A13 (14.0962, 32.3404) -> (17.5486, 28.2182) centre (15.8224, 30.2793) ccw
  arc A14 (28.2966, 28.2182) -> (17.5486, 28.2182) centre (22.9226, 21.8016) ccw
  spline S42 degree 2 poles (17.1059, 31.3027) (17.4052, 31.4869) (17.5047, 31.7133) knots 0 0 0 1 1 1
  spline S43 degree 2 poles (17.5047, 31.7133) (17.6062, 31.9409) (17.4141, 32.253) knots 0 0 0 1 1 1
  spline S44 degree 2 poles (17.4141, 32.253) (17.2074, 32.5886) (16.8887, 32.5604) knots 0 0 0 1 1 1
  spline S45 degree 2 poles (16.8887, 32.5604) (16.7188, 32.5443) (16.5008, 32.41) knots 0 0 0 1 1 1
  line L55 (16.5008, 32.41) -> (15.4618, 31.7704)
  line L56 (15.4618, 31.7704) -> (16.1226, 30.6972)
  line L57 (16.1226, 30.6972) -> (17.1059, 31.3027)
  line L58 (14.8114, 31.874) -> (16.265, 32.769)
  spline S46 degree 2 poles (16.265, 32.769) (16.6242, 32.9901) (16.9217, 33.0288) knots 0 0 0 1 1 1
  spline S47 degree 2 poles (16.9217, 33.0288) (17.4879, 33.1004) (17.8209, 32.5595) knots 0 0 0 1 1 1
  spline S48 degree 2 poles (17.8209, 32.5595) (17.9946, 32.2773) (17.9876, 32.0254) knots 0 0 0 1 1 1
  spline S49 degree 2 poles (17.9876, 32.0254) (17.9827, 31.7747) (17.8404, 31.5367) knots 0 0 0 1 1 1
  spline S50 degree 2 poles (17.8404, 31.5367) (18.0703, 31.5751) (18.2372, 31.5098) knots 0 0 0 1 1 1
  spline S51 degree 2 poles (18.2372, 31.5098) (18.4063, 31.4459) (18.5855, 31.1789) knots 0 0 0 1 1 1
  line L59 (18.5855, 31.1789) -> (18.8597, 30.7669)
  spline S52 degree 2 poles (18.8597, 30.7669) (18.9767, 30.5913) (19.0542, 30.5182) knots 0 0 0 1 1 1
  spline S53 degree 2 poles (19.0542, 30.5182) (19.1848, 30.3922) (19.3095, 30.41) knots 0 0 0 1 1 1
  line L60 (19.3095, 30.41) -> (19.3529, 30.3395)
  line L61 (19.3529, 30.3395) -> (18.8313, 30.0183)
  spline S54 degree 2 poles (18.8313, 30.0183) (18.7849, 30.0458) (18.7326, 30.102) knots 0 0 0 1 1 1
  spline S55 degree 2 poles (18.7326, 30.102) (18.6803, 30.1582) (18.5585, 30.3368) knots 0 0 0 1 1 1
  line L62 (18.5585, 30.3368) -> (18.2104, 30.8447)
  spline S56 degree 2 poles (18.2104, 30.8447) (18.0059, 31.1434) (17.7277, 31.1165) knots 0 0 0 1 1 1
  spline S57 degree 2 poles (17.7277, 31.1165) (17.5703, 31.0992) (17.3095, 30.9386) knots 0 0 0 1 1 1
  line L63 (17.3095, 30.9386) -> (16.3411, 30.3424)
  line L64 (16.3411, 30.3424) -> (17.1703, 28.9956)
  line L65 (17.1703, 28.9956) -> (16.7449, 28.7337)
  line L66 (16.7449, 28.7337) -> (14.8114, 31.874)
  line L67 (21.5319, 32.3468) -> (20.6778, 33.8429)
  line L68 (20.6778, 33.8429) -> (20.3974, 32.1313)
  line L69 (20.3974, 32.1313) -> (21.5319, 32.3468)
  line L70 (20.3192, 34.3319) -> (20.8741, 34.4373)
  line L71 (20.8741, 34.4373) -> (22.8769, 31.064)
  line L72 (22.8769, 31.064) -> (22.3392, 30.9619)
  line L73 (22.3392, 30.9619) -> (21.7656, 31.9772)
  line L74 (21.7656, 31.9772) -> (20.3327, 31.705)
  line L75 (20.3327, 31.705) -> (20.1467, 30.5453)
  line L76 (20.1467, 30.5453) -> (19.6436, 30.4498)
  line L77 (19.6436, 30.4498) -> (20.3192, 34.3319)
  line L78 (24.0048, 34.6669) -> (24.5859, 34.5651)
  line L79 (24.5859, 34.5651) -> (25.9049, 31.3009)
  line L80 (25.9049, 31.3009) -> (26.4206, 34.2435)
  line L81 (26.4206, 34.2435) -> (26.888, 34.1616)
  line L82 (26.888, 34.1616) -> (26.2513, 30.5291)
  line L83 (26.2513, 30.5291) -> (25.6999, 30.6258)
  line L84 (25.6999, 30.6258) -> (24.3532, 33.8922)
  line L85 (24.3532, 33.8922) -> (23.8379, 30.9521)
  line L86 (23.8379, 30.9521) -> (23.3681, 31.0345)
  line L87 (23.3681, 31.0345) -> (24.0048, 34.6669)
  spline S58 degree 2 poles (28.446, 29.8605) (28.6619, 29.7276) (28.8285, 29.6869) knots 0 0 0 1 1 1
  spline S59 degree 2 poles (28.8285, 29.6869) (29.1278, 29.6176) (29.4321, 29.7575) knots 0 0 0 1 1 1
  spline S60 degree 2 poles (29.4321, 29.7575) (29.6753, 29.8701) (29.9139, 30.133) knots 0 0 0 1 1 1
  spline S61 degree 2 poles (29.9139, 30.133) (30.0552, 30.2907) (30.1486, 30.4425) knots 0 0 0 1 1 1
  spline S62 degree 2 poles (30.1486, 30.4425) (30.508, 31.0261) (30.4737, 31.4923) knots 0 0 0 1 1 1
  spline S63 degree 2 poles (30.4737, 31.4923) (30.4416, 31.9573) (29.9264, 32.2745) knots 0 0 0 1 1 1
  line L88 (29.9264, 32.2745) -> (29.1718, 32.7391)
  line L89 (29.1718, 32.7391) -> (27.6871, 30.3277)
  line L90 (27.6871, 30.3277) -> (28.446, 29.8605)
  line L91 (28.9693, 33.3679) -> (30.2412, 32.5847)
  spline S64 degree 2 poles (30.2412, 32.5847) (30.889, 32.1859) (30.963, 31.5065) knots 0 0 0 1 1 1
  spline S65 degree 2 poles (30.963, 31.5065) (31.0262, 30.8957) (30.6273, 30.2479) knots 0 0 0 1 1 1
  spline S66 degree 2 poles (30.6273, 30.2479) (30.3193, 29.7477) (29.8825, 29.4595) knots 0 0 0 1 1 1
  spline S67 degree 2 poles (29.8825, 29.4595) (29.1115, 28.9495) (28.3034, 29.4471) knots 0 0 0 1 1 1
  line L92 (28.3034, 29.4471) -> (27.0358, 30.2276)
  line L93 (27.0358, 30.2276) -> (28.9693, 33.3679)
  arc A15 (8.8654, 39.6892) -> (-8.7873, 39.6892) centre (0.039, 29.1504) ccw
  arc A16 (-8.7873, 39.6892) -> (-5.335, 35.567) centre (-7.0611, 37.6281) ccw
  arc A17 (5.4131, 35.567) -> (-5.335, 35.567) centre (0.039, 29.1504) ccw
  arc A18 (5.4131, 35.567) -> (8.8654, 39.6892) centre (7.1392, 37.6281) ccw
  line L94 (-7.9264, 39.6594) -> (-7.4554, 39.9169)
  line L95 (-7.4554, 39.9169) -> (-5.7812, 36.8541)
  line L96 (-5.7812, 36.8541) -> (-4.0202, 37.8167)
  line L97 (-4.0202, 37.8167) -> (-3.7938, 37.4024)
  line L98 (-3.7938, 37.4024) -> (-6.0258, 36.1824)
  line L99 (-6.0258, 36.1824) -> (-7.9264, 39.6594)
  line L100 (-1.9966, 41.9387) -> (-1.2279, 41.943)
  line L101 (-1.2279, 41.943) -> (-0.0708, 38.5992)
  line L102 (-0.0708, 38.5992) -> (1.0407, 41.9557)
  line L103 (1.0407, 41.9557) -> (1.8013, 41.96)
  line L104 (1.8013, 41.96) -> (1.8235, 37.9975)
  line L105 (1.8235, 37.9975) -> (1.3137, 37.9946)
  line L106 (1.3137, 37.9946) -> (1.3006, 40.3333)
  spline S68 degree 2 poles (1.3006, 40.3333) (1.2999, 40.4547) (1.3038, 40.7352) knots 0 0 0 1 1 1
  spline S69 degree 2 poles (1.3038, 40.7352) (1.3076, 41.0158) (1.3058, 41.3368) knots 0 0 0 1 1 1
  line L107 (1.3058, 41.3368) -> (0.1943, 37.9884)
  line L108 (0.1943, 37.9884) -> (-0.3371, 37.9854)
  line L109 (-0.3371, 37.9854) -> (-1.4941, 41.3211)
  line L110 (-1.4941, 41.3211) -> (-1.4935, 41.1997)
  spline S70 degree 2 poles (-1.4935, 41.1997) (-1.4926, 41.0541) (-1.4856, 40.7547) knots 0 0 0 1 1 1
  spline S71 degree 2 poles (-1.4856, 40.7547) (-1.4758, 40.458) (-1.475, 40.3178) knots 0 0 0 1 1 1
  line L111 (-1.475, 40.3178) -> (-1.4619, 37.9791)
  line L112 (-1.4619, 37.9791) -> (-1.9745, 37.9762)
  line L113 (-1.9745, 37.9762) -> (-1.9966, 41.9387)
  spline S72 degree 2 poles (6.815, 38.1522) (7.1378, 37.9563) (7.403, 37.9721) knots 0 0 0 1 1 1
  spline S73 degree 2 poles (7.403, 37.9721) (7.6705, 37.9864) (7.8748, 38.3231) knots 0 0 0 1 1 1
  spline S74 degree 2 poles (7.8748, 38.3231) (8.0945, 38.6852) (7.9114, 38.9761) knots 0 0 0 1 1 1
  spline S75 degree 2 poles (7.9114, 38.9761) (7.8127, 39.1307) (7.5775, 39.2735) knots 0 0 0 1 1 1
  line L114 (7.5775, 39.2735) -> (6.4568, 39.9536)
  line L115 (6.4568, 39.9536) -> (5.7543, 38.796)
  line L116 (5.7543, 38.796) -> (6.815, 38.1522)
  line L117 (6.2373, 40.6265) -> (7.8053, 39.6748)
  spline S76 degree 2 poles (7.8053, 39.6748) (8.1927, 39.4396) (8.3755, 39.1741) knots 0 0 0 1 1 1
  spline S77 degree 2 poles (8.3755, 39.1741) (8.7213, 38.6676) (8.3672, 38.0842) knots 0 0 0 1 1 1
  spline S78 degree 2 poles (8.3672, 38.0842) (8.1824, 37.7798) (7.9381, 37.6631) knots 0 0 0 1 1 1
  spline S79 degree 2 poles (7.9381, 37.6631) (7.696, 37.545) (7.3986, 37.5645) knots 0 0 0 1 1 1
  spline S80 degree 2 poles (7.3986, 37.5645) (7.5479, 37.3635) (7.5673, 37.1718) knots 0 0 0 1 1 1
  spline S81 degree 2 poles (7.5673, 37.1718) (7.589, 36.9788) (7.4214, 36.6766) knots 0 0 0 1 1 1
  line L118 (7.4214, 36.6766) -> (7.1618, 36.2126)
  spline S82 degree 2 poles (7.1618, 36.2126) (7.0512, 36.0147) (7.0192, 35.9047) knots 0 0 0 1 1 1
  spline S83 degree 2 poles (7.0192, 35.9047) (6.9627, 35.7181) (7.0408, 35.6076) knots 0 0 0 1 1 1
  line L119 (7.0408, 35.6076) -> (6.9946, 35.5315)
  line L120 (6.9946, 35.5315) -> (6.4319, 35.873)
  spline S84 degree 2 poles (6.4319, 35.873) (6.4354, 35.9308) (6.4636, 36.0084) knots 0 0 0 1 1 1
  spline S85 degree 2 poles (6.4636, 36.0084) (6.4918, 36.086) (6.6029, 36.2899) knots 0 0 0 1 1 1
  line L121 (6.6029, 36.2899) -> (6.9181, 36.8717)
  spline S86 degree 2 poles (6.9181, 36.8717) (7.1035, 37.2135) (6.9415, 37.4665) knots 0 0 0 1 1 1
  spline S87 degree 2 poles (6.9415, 37.4665) (6.8479, 37.6085) (6.5665, 37.7792) knots 0 0 0 1 1 1
  line L122 (6.5665, 37.7792) -> (5.5219, 38.4132)
  line L123 (5.5219, 38.4132) -> (4.6402, 36.9605)
  line L124 (4.6402, 36.9605) -> (4.1813, 37.239)
  line L125 (4.1813, 37.239) -> (6.2373, 40.6265)
  point P0 (-23, 21.8016)
  dimension "d61" = 15
  dimension "d62" = 15
  constraint coincident P0 A4.centre
  constraint tangent A6 A7
  constraint tangent A7 A8
  constraint tangent A8 A9
  constraint tangent A6 A9
  constraint coincident A5.centre A6.centre
  constraint horizontal A9.centre A7.centre
  constraint tangent A11 A12
  constraint tangent A11 A14
  constraint tangent A13 A14
  constraint tangent A12 A13
  constraint horizontal A13.centre A11.centre
  constraint tangent A15 A18
  constraint tangent A17 A18
  constraint tangent A16 A17
  constraint tangent A15 A16
  constraint horizontal A16.centre A18.centre
  measures "d61" diameter of A4
  measures "d62" diameter of A5
extrude "Extrude4'" add sketch "Sketch1 (2)" along normal blind 2 separate body contours S0 S1 S2 S3 S4 S5 L13 S6 S7 S8 S9 S10 S11 L14 S12 S13 S14 S15 S16 S17 L15 S18 S19 S20 S21 S22 S23 L16 | L17 S24 S25 S26 S27 L18 L19 L20 L21 | L25 L26 L27 L28 L29 L30 L31 L32 L33 L34 L35 L36 | L37 L38 L39 L40 L41 L42 L43 L44 L45 L46 L47 L48 | L52 S38 S39 S40 S41 L53 L54 | L58 S46 S47 S48 S49 S50 S51 L59 S52 S53 L60 L61 S54 S55 L62 S56 S57 L63 L64 L65 L66 | L70 L71 L72 L73 L74 L75 L76 L77 | L78 L79 L80 L81 L82 L83 L84 L85 L86 L87 | L91 S64 S65 S66 S67 L92 L93 | L94 L95 L96 L97 L98 L99 | L100 L101 L102 L103 L104 L105 L106 S68 S69 L107 L108 L109 L110 S70 S71 L111 L112 L113 | L117 S76 S77 S78 S79 S80 S81 L118 S82 S83 L119 L120 S84 S85 L121 S86 S87 L122 L123 L124 L125 makes body 3 at (19.8688, -35.6667, 31.7438) makes body 4 at (-24.3361, -35.6667, 32.3496) makes body 5 at (-27.4905, -35.6667, 31.3647) makes body 6 at (16.1004, -35.6667, 29.7804) makes body 7 at (26.6757, -35.6667, 32.9507) makes body 8 at (-21.0345, -35.6667, 32.2023) makes body 9 at (-29.5083, -35, 30.6576) makes body 10 at (-17.9772, -35.6667, 30.9501) makes body 11 at (27.6803, -35.6667, 31.2743) makes body 12 at (-6.6593, -35.6667, 37.3414) makes body 13 at (1.8087, -35.6667, 40.6391) makes body 14 at (4.8666, -35.6667, 38.3682) in component "dials"
extrude "Extrude5'" add sketch "Sketch1 (2)" along normal blind 1 contours A6 A7 A8 A9 | S28 S29 L22 L23 L24 S30 S31 | S32 S33 S34 S35 S36 S37 L49 L50 L51 | A11 A12 A13 A14 | S42 S43 S44 S45 L55 L56 L57 | L67 L68 L69 | S58 S59 S60 S61 S62 S63 L88 L89 L90 | A15 A16 A17 A18 | S72 S73 S74 S75 L114 L115 L116 bodies 12 4 3 13 14 5 6 7 8 9 10 11 in component "dials"
component "base" placed x (1, 0, 0) y (0, 1, 0) z (0, 0, 1) at (0, 0, 0)
component "dials" placed x (1, 0, 0) y (0, 1, 0) z (0, 0, 1) at (0, 0, 0)
